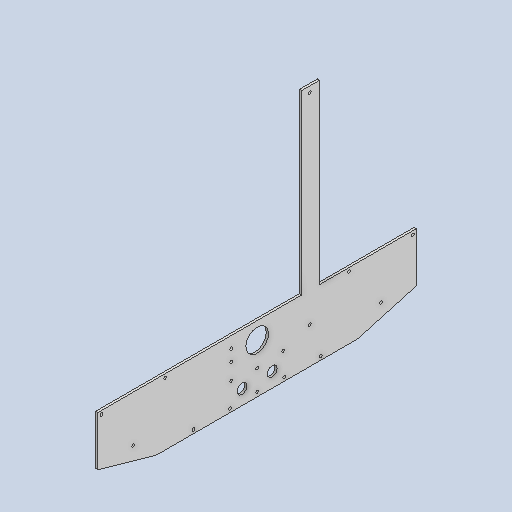
# Autodesk Inventor part: Outside Chassi Plate low
Saved by Autodesk Inventor 2023 (Build 270158000, 158)
## iProperties
Created: 2022-09-05
Part Number: Outside Chassi Plate low
Material: Generic
Document SubType Name: Modeling
Designer: deli
Density: 1 g/cm^3
Appearance: Default
Author: deli
Autodesk Inventor part; units mm, degrees
ref_plane "YZ Plane" through (0, 0, 0) normal (1, 0, 0) x (0, 1, 0)
ref_plane "XZ Plane" through (0, 0, 0) normal (0, 1, 0) x (-1, 0, 0)
ref_plane "XY Plane" through (0, 0, 0) normal (0, 0, 1) x (1, 0, 0)
sketch "Sketch1" plane through (0, 0, 0) normal (1, 0, 0) x (0, 1, 0)
  line L0 (-213.0456, 506.9498) -> (-283.0456, 506.9498)
  line L1 (-283.0456, 506.9498) -> (-306.2682, 424.6818)
  line L2 (-213.0456, 56.9498) -> (-283.0456, 56.9498)
  circle A0 centre (-278.4562, 456.9498) radius 2
  circle A1 centre (-278.4562, 456.9498) radius 48 construction
  arc A2 (-266.5301, 456.4491) -> (-290.3765, 457.5739) centre (-278.4562, 456.9498) ccw construction
  circle A3 centre (-278.4562, 106.9498) radius 48 construction
  arc A4 (-290.3765, 106.3258) -> (-266.5301, 107.4505) centre (-278.4562, 106.9498) ccw construction
  circle A5 centre (-278.4562, 106.9498) radius 2
  circle A6 centre (-285.7062, 303.2411) radius 7
  circle A7 centre (-285.7062, 260.6586) radius 7
  circle A8 centre (-285.7062, 303.2411) radius 18.75 construction
  circle A9 centre (-285.7062, 260.6586) radius 18.75 construction
  arc A10 (-298.4212, 303.9067) -> (-272.985, 302.707) centre (-285.7062, 303.2411) ccw construction
  arc A11 (-272.985, 261.1927) -> (-298.4212, 259.9929) centre (-285.7062, 260.6586) ccw construction
  line L3 (-266.5301, 456.4491) -> (-272.985, 302.707) construction
  line L4 (-298.4212, 303.9067) -> (-290.3765, 457.5739) construction
  line L5 (-272.985, 261.1927) -> (-266.5301, 107.4505) construction
  line L6 (-290.3765, 106.3258) -> (-298.4212, 259.9929) construction
  circle A12 centre (-271.2236, 281.9498) radius 2
  circle A13 centre (-300.1888, 281.9498) radius 2
  circle A14 centre (-301.4562, 320.3437) radius 2
  circle A15 centre (-301.4562, 243.5559) radius 2
  circle A16 centre (-268.3114, 245.2319) radius 2
  circle A17 centre (-218.0456, 501.9498) radius 2
  circle A18 centre (-218.0456, 61.9498) radius 2
  arc A19 (-306.4562, 229.9036) -> (-306.4562, 229.9036) centre (-283.7062, 229.9036) ccw
  line L7 (-306.4562, 189.1468) -> (-306.4562, 229.9036)
  arc A20 (-306.4562, 189.1468) -> (-306.4562, 189.1468) centre (-283.7062, 189.1468) ccw
  arc A21 (-306.2682, 424.6818) -> (-306.4562, 423.3235) centre (-301.4562, 423.3235) ccw
  line L8 (-306.4562, 423.3235) -> (-306.4562, 229.9036)
  line L9 (-283.0456, 56.9498) -> (-306.2682, 139.2178)
  line L10 (-306.4562, 189.1468) -> (-306.4562, 140.5761)
  circle A22 centre (-268.3114, 318.6677) radius 2
  arc A23 (-306.4562, 140.5761) -> (-306.2682, 139.2178) centre (-301.4562, 140.5761) ccw
  circle A24 centre (-218.0456, 411.9498) radius 2
  circle A25 centre (-218.0456, 151.9498) radius 2
  circle A26 centre (-301.4562, 371.8336) radius 2
  line L11 (36.9544, 193.3998) -> (-213.0456, 193.3998)
  line L12 (-213.0456, 218.7998) -> (36.9544, 218.7998)
  line L13 (36.9544, 218.7998) -> (36.9544, 193.3998)
  line L14 (-213.0456, 506.9498) -> (-213.0456, 218.7998)
  line L15 (-213.0456, 193.3998) -> (-213.0456, 56.9498)
  line L16 (-263.0456, 193.3998) -> (36.9544, 193.3998) construction
  circle A27 centre (20.9544, 281.9498) radius 5 construction
  line L17 (-263.0456, 193.3998) -> (36.9544, 193.3998) construction
  circle A28 centre (20.9544, 281.9498) radius 5 construction
  circle A29 centre (28.9544, 207.6873) radius 2
  circle A30 centre (-255.0456, 207.6873) radius 2
  line L18 (-213.0456, 314.4098) -> (-261.0456, 314.4098) construction
  line L19 (-261.0456, 314.4098) -> (-261.0456, 326.4098) construction
  line L20 (-261.0456, 326.4098) -> (-213.0456, 326.4098) construction
  line L21 (-213.0456, 326.4098) -> (-213.0456, 314.4098) construction
  line L22 (-216.0456, 326.4098) -> (-258.0456, 326.4098) construction
  line L23 (-258.0456, 326.4098) -> (-258.0456, 330.4098) construction
  line L24 (-258.0456, 330.4098) -> (-216.0456, 330.4098) construction
  line L25 (-216.0456, 330.4098) -> (-216.0456, 326.4098) construction
  line L26 (-233.0456, 326.4098) -> (-241.0456, 326.4098) construction
  line L27 (-241.0456, 326.4098) -> (-241.0456, 294.4098) construction
  line L28 (-241.0456, 294.4098) -> (-233.0456, 294.4098) construction
  line L29 (-233.0456, 294.4098) -> (-233.0456, 326.4098) construction
  line L30 (-218.2956, 330.4098) -> (-255.7956, 330.4098) construction
  line L31 (-255.7956, 330.4098) -> (-255.7956, 405.4098) construction
  line L32 (-255.7956, 405.4098) -> (-218.2956, 405.4098) construction
  line L33 (-218.2956, 405.4098) -> (-218.2956, 330.4098) construction
  line L34 (-213.0456, 323.9098) -> (-261.0456, 323.9098) construction
  line L35 (-217.0456, 323.9098) -> (-257.0456, 323.9098) construction
  line L36 (-257.0456, 323.9098) -> (-257.0456, 320.9098) construction
  line L37 (-257.0456, 320.9098) -> (-217.0456, 320.9098) construction
  line L38 (-217.0456, 320.9098) -> (-217.0456, 323.9098) construction
  line L39 (-227.5456, 320.9098) -> (-246.5456, 320.9098) construction
  line L40 (-246.5456, 320.9098) -> (-246.5456, 317.9098) construction
  line L41 (-246.5456, 317.9098) -> (-227.5456, 317.9098) construction
  line L42 (-227.5456, 317.9098) -> (-227.5456, 320.9098) construction
  line L43 (-229.2956, 317.9098) -> (-244.7956, 317.9098) construction
  line L44 (-244.7956, 317.9098) -> (-244.7956, 312.9498) construction
  line L45 (-244.7956, 312.9498) -> (-229.2956, 312.9498) construction
  line L46 (-229.2956, 312.9498) -> (-229.2956, 317.9098) construction
  line L47 (-227.6956, 312.9498) -> (-246.3956, 312.9498) construction
  line L48 (-246.3956, 312.9498) -> (-246.3956, 303.4498) construction
  line L49 (-246.3956, 303.4498) -> (-227.6956, 303.4498) construction
  line L50 (-227.6956, 303.4498) -> (-227.6956, 312.9498) construction
  line L51 (-249.0456, 303.4498) -> (-225.0456, 303.4498) construction
  line L52 (-225.0456, 303.4498) -> (-225.0456, 298.4498) construction
  line L53 (-225.0456, 298.4498) -> (-249.0456, 298.4498) construction
  line L54 (-249.0456, 298.4498) -> (-249.0456, 303.4498) construction
  circle A31 centre (-237.0456, 281.9498) radius 16
  circle A32 centre (-301.4562, 192.066) radius 2
  circle A33 centre (-229.0456, 318.4098) radius 2
  circle A34 centre (-245.0456, 318.4098) radius 2
  point P0 (0, 0)
  point P1 (-213.0456, 320.4098)
  dimension "d43" = 450
  dimension "d44" = 4
  dimension "d46" = 96
  dimension "d47" = 23.8732
  dimension "d48" = 96
  dimension "d49" = 4
  dimension "d51" = 23.8732
  dimension "d54" = 50
  dimension "d55" = 50
  dimension "d56" = 70
  dimension "d57" = 70
  dimension "d58" = 14
  dimension "d59" = 14
  dimension "d60" = 37.5
  dimension "d61" = 37.5
  dimension "d62" = 25.4648
  dimension "d63" = 25.4648
  dimension "d64" = 179.407
  dimension "d65" = 179.407
  dimension "d66" = 179.407
  dimension "d67" = 179.407
  dimension "d68" = 153.8776
  dimension "d70" = 153.8776
  dimension "d74" = 4
  dimension "d75" = 4
  dimension "d77" = 4
  dimension "d78" = 4
  dimension "d91" = 5
  dimension "d92" = 5
  dimension "d94" = 2.5
  dimension "d95" = 2.5
  dimension "d97" = 2.5
  dimension "d103" = 4
  dimension "d106" = 4
  dimension "d108" = 5
  dimension "d112" = 5
  dimension "d120" = 4
  dimension "d124" = 28
  dimension "d125" = 20.75
  dimension "d127" = 20.75
  dimension "d142" = 4
  dimension "d143" = 2.5
  dimension "d144" = 4
  dimension "d145" = 4
  dimension "d146" = 18
  dimension "d147" = 18
  dimension "d148" = 5
  dimension "d149" = 5
  dimension "d150" = 440
  dimension "d151" = 4
  dimension "d153" = 4
  dimension "d154" = 4
  dimension "d157" = 5
  dimension "d161" = 90
  dimension "d166" = 5
  dimension "d167" = 5
  dimension "d174" = 5
  dimension "d175" = 5
  dimension "d176" = 25.4
  dimension "d177" = 88.55
  dimension "d178" = 136.45
  dimension "d179" = 4
  dimension "d180" = 4
  dimension "d181" = 11.1125
  constraints: 106 end point, 33 centre point, 19 parallel, 17 point on circle, 16 tangent, 14 perpendicular, 11 horizontal, 10 point on line, 7 vertical, 6 coincident, 2 concentric, 1 midpoint
  measures "d43" distance of L0.start L2.start
  measures "d44" diameter of A0
  measures "d46" diameter of A1
  measures "d47" diameter of A2
  measures "d48" diameter of A3
  measures "d49" diameter of A5
  measures "d51" diameter of A4
  measures "d54" distance from line of A0.centre L0
  measures "d55" distance from line of L2 A5.centre
  measures "d56" distance of L0.start L0.end
  measures "d57" distance of L2.start L2.end
  measures "d58" diameter of A6
  measures "d59" diameter of A7
  measures "d60" diameter of A8
  measures "d61" diameter of A9
  measures "d62" diameter of A10
  measures "d63" diameter of A11
  measures "d68" distance of L3.start L3.end
  measures "d70" distance of L5.start L5.end
  measures "d74" diameter of A14
  measures "d75" diameter of A13
  measures "d77" diameter of A12
  measures "d78" diameter of A16
  measures "d103" diameter of A17
  measures "d106" diameter of A18
  measures "d108" distance from line of L0 A17.centre
  measures "d112" distance from line of L2 A18.centre
  measures "d120" diameter of A15
  measures "d124" distance from line of A0.centre L7
  measures "d125" distance from line of L7 A6.centre
  measures "d127" distance from line of L7 A7.centre
  measures "d142" distance from line of L5 A16.centre
  measures "d144" distance from line of L3 A22.centre
  measures "d145" diameter of A22
  measures "d146" distance from line of A0.centre L1
  measures "d147" distance from line of L9 A3.centre
  measures "d148" radius of A21
  measures "d149" radius of A23
  measures "d150" distance of A18.centre A17.centre
  measures "d151" diameter of A24
  measures "d153" diameter of A25
  measures "d154" diameter of A26
  measures "d157" distance from line of L8 A26.centre
  measures "d161" distance of A24.centre A17.centre
  measures "d166" distance from line of L8 A14.centre
  measures "d167" distance from line of L10 A15.centre
  measures "d176" distance of L12.end L11.start
  measures "d177" distance from line of A27.centre L16
  measures "d178" distance between parallel lines of L11 L2
  measures "d179" diameter of A30
  measures "d180" diameter of A29
  measures "d181" distance from line of L12 A29.centre
extrude "Extrusion1" add sketch "Sketch1" along normal blind 3.175 contours L14 L12 L13 L11 L15 L2 L9 A23 L10 A20 A19 A16 A15 L8 A21 L1 L0 | A19 A15 A16 A20 | A19 A20 L7 | A20 A19 | A19 A20
body "Solid1"
